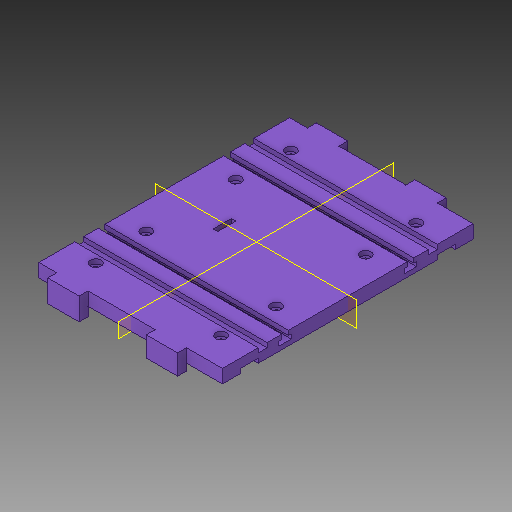
# Autodesk Inventor part: BandSawJigBottom
Saved by Autodesk Inventor 2019 (Build 230136000, 136)
## iProperties
Created: 2017-12-10
Part Number: BandSawJigBottom
Material: LCP Plastic
Document SubType Name: Modeling
Designer: steele
Density: 1.626 g/cm^3
Appearance: Violet
Author: steele
Autodesk Inventor part; units mm, degrees
ref_plane "YZ Plane" through (0, 0, 0) normal (1, 0, 0) x (0, 1, 0)
ref_plane "XZ Plane" through (0, 0, 0) normal (0, 1, 0) x (-1, 0, 0)
sketch "Sketch3" plane through (0, 0, 0) normal (0, 0, 1) x (1, 0, 0)
  line L0 (0, -9.525) -> (9.525, -9.525)
  line L1 (9.525, -9.525) -> (9.525, 0)
  line L2 (0, 0) -> (0, -9.525) construction
  line L3 (0, 0) -> (9.525, 0) construction
  line L4 (0, -9.525) -> (-9.525, -9.525)
  line L5 (-9.525, -9.525) -> (-9.525, 0)
  line L6 (9.525, 0) -> (73.025, 0)
  line L7 (-187.325, 0) -> (-187.325, 19.05)
  line L8 (-187.325, 0) -> (-9.525, 0)
  line L9 (73.025, 0) -> (73.025, 19.05)
  line L10 (73.025, 19.05) -> (-187.325, 19.05)
  dimension "d0" = 9.525
  dimension "d1" = 9.525
  dimension "d6" = 63.5
  dimension "d8" = 19.05
  dimension "d9" = 177.8
  constraints: 22 end point, 4 horizontal, 3 perpendicular, 2 symmetric about line, 1 vertical
  measures "d0" distance of L0.end L1.end
  measures "d1" distance of L0.start L0.end
  measures "d6" distance of L1.end L6.end
  measures "d8" distance of L6.end L9.end
  measures "d9" distance of L7.start L5.end
extrude "Extrusion1" add sketch "Sketch3" along normal mid plane 355.6
sketch "Sketch4" plane through (0, 0, 177.8) normal (0, 0, 1) x (1, 0, 0)
  line L0 (-187.325, 19.05) -> (73.025, 19.05) construction
  line L1 (0, 19.05) -> (0, -9.525) construction
  line L2 (9.525, -9.525) -> (-9.525, -9.525) construction
  line L3 (0, -9.525) -> (-22.225, -9.525)
  line L4 (-22.225, -9.525) -> (-22.225, 19.05)
  line L5 (-22.225, 19.05) -> (0, 19.05)
  line L6 (187.325, 19.05) -> (-73.025, 19.05) construction
  line L7 (0, -9.525) -> (22.225, -9.525)
  line L8 (22.225, -9.525) -> (22.225, 19.05)
  line L9 (0, 19.05) -> (22.225, 19.05)
  point P0 (0, 0)
  dimension "d12" = 22.225
  constraints: 16 end point, 4 point on line, 4 symmetric about line, 2 collinear, 1 midpoint, 1 perpendicular
  measures "d12" distance of L1.end L3.end
extrude "Extrusion2" add sketch "Sketch4" along normal blind 12.7
mirror "Mirror1" about plane through (0, 0, 0) normal (0, 0, 1) of "Extrusion2"
sketch "Sketch6" plane through (-187.325, 0, -177.8) normal (0, -1, 0) x (1, 0, 0)
  line L0 (82.55, 165.1) -> (88.9, 165.1)
  line L1 (88.9, 165.1) -> (88.9, 190.5)
  line L2 (88.9, 190.5) -> (82.55, 190.5)
  line L3 (82.55, 190.5) -> (82.55, 165.1)
  line L4 (82.55, 165.1) -> (88.9, 190.5) construction
  line L5 (88.9, 165.1) -> (82.55, 190.5) construction
  line L6 (177.8, 0) -> (177.8, 355.6) projected
  point P0 (187.325, 177.8)
  point P1 (85.725, 177.8)
  dimension "d16" = 12.7
  dimension "d18" = 6.35
  dimension "d19" = 88.9
  constraints: 12 end point, 2 midpoint, 2 parallel, 1 horizontal, 1 perpendicular
  measures "d16" distance from line of L2 point (85.725, 177.8)
  measures "d18" distance of L1.end L2.end
  measures "d19" distance between parallel lines of L1 L6
extrude "Extrusion3" cut sketch "Sketch6" against normal through all
sketch "Sketch7" plane through (0, 0, 177.8) normal (0, 0, 1) x (1, 0, 0)
  line L0 (-187.325, 19.05) -> (-22.225, 19.05) projected
  line L1 (-161.925, 19.05) -> (-117.475, 19.05)
  line L2 (-117.475, 19.05) -> (-117.475, -12.7)
  line L3 (-117.475, -12.7) -> (-161.925, -12.7)
  line L4 (-161.925, -12.7) -> (-161.925, 19.05)
  line L5 (-187.325, 19.05) -> (-187.325, 0) projected
  point P0 (0, 0)
  dimension "d22" = 44.45
  dimension "d23" = 31.75
  dimension "d24" = 25.4
  constraints: 8 end point, 2 parallel, 1 horizontal, 1 perpendicular, 1 point on line
  measures "d22" distance of L2.end L3.end
  measures "d23" distance of L1.end L2.end
  measures "d24" distance between parallel lines of L4 L5
extrude "Extrusion4" add sketch "Sketch7" along normal blind 12.7
mirror "Mirror2" about plane through (0, 0, 0) normal (0, 0, 1) of "Extrusion4"
sketch "Sketch9" plane through (73.025, 0, 177.8) normal (1, 0, 0) x (0, 0, -1)
  line L0 (355.6, 19.05) -> (0, 19.05) projected
  line L1 (50.8, 19.05) -> (63.5, 19.05)
  line L2 (63.5, 19.05) -> (63.5, 12.7)
  line L3 (63.5, 12.7) -> (50.8, 12.7)
  line L4 (50.8, 12.7) -> (50.8, 19.05)
  line L5 (0, 0) -> (0, 19.05) projected
  point P0 (177.8, 0)
  dimension "d28" = 12.7
  dimension "d29" = 6.35
  dimension "d30" = 50.8
  constraints: 8 end point, 2 parallel, 1 horizontal, 1 perpendicular, 1 point on line
  measures "d28" distance of L2.end L3.end
  measures "d29" distance of L1.end L2.end
  measures "d30" distance between parallel lines of L4 L5
extrude "Extrusion5" cut sketch "Sketch9" against normal through all
mirror "Mirror3" about plane through (0, 0, 0) normal (0, 0, 1) of "Extrusion5"
sketch "Sketch12" plane through (73.025, 0, 177.8) normal (1, 0, 0) x (0, 0, -1)
  line L0 (355.6, 0) -> (0, 0) construction
  line L1 (88.9, 0) -> (88.9, 16.5009) construction
  line L2 (0, 0) -> (0, 19.05) projected
  line L3 (50.8, 19.05) -> (0, 19.05) projected
  line L4 (84.1375, 19.05) -> (84.1375, 12.7)
  line L5 (84.1375, 12.7) -> (80.1624, 12.7)
  line L6 (80.1624, 12.7) -> (80.1624, 6.35)
  line L7 (80.1624, 6.35) -> (88.9, 6.35)
  line L8 (93.6625, 19.05) -> (93.6625, 12.7)
  line L9 (93.6625, 12.7) -> (97.6376, 12.7)
  line L10 (97.6376, 12.7) -> (97.6376, 6.35)
  line L11 (97.6376, 6.35) -> (88.9, 6.35)
  line L12 (84.1375, 19.05) -> (93.6625, 19.05)
  point P0 (177.8, 0)
  dimension "d46" = 88.9
  dimension "d47" = 4.7625
  dimension "d48" = 6.35
  dimension "d49" = 6.35
  dimension "d50" = 8.7376
  constraints: 20 end point, 4 symmetric about line, 3 point on line, 3 vertical, 1 collinear, 1 horizontal, 1 perpendicular
  measures "d46" distance between parallel lines of L1 L2
  measures "d47" distance between parallel lines of L4 L1
  measures "d48" distance of L4.start L4.end
  measures "d49" distance of L5.end L6.end
  measures "d50" distance of L6.end L7.end
extrude "Extrusion8" cut sketch "Sketch12" against normal through all
mirror "Mirror4" about plane through (0, 0, 0) normal (0, 0, 1) of "Extrusion8"
ref_plane "Work Plane1" through (-57.15, 0, 177.8) normal (1, 0, 0) x (0, 0, -1)
sketch "Sketch13" plane through (-57.15, 0, 177.8) normal (1, 0, 0) x (0, 0, -1)
  line L0 (25.4, 0) -> (50.8, 0)
  line L1 (50.8, 0) -> (50.8, 6.35)
  line L2 (50.8, 6.35) -> (25.4, 6.35)
  line L3 (25.4, 6.35) -> (25.4, 0)
  line L4 (0, 0) -> (0, 19.05) projected
  point P0 (177.8, 0)
  dimension "d54" = 25.4
  dimension "d55" = 6.35
  dimension "d56" = 25.4
  constraints: 8 end point, 2 parallel, 1 horizontal, 1 perpendicular
  measures "d54" distance of L0.start L0.end
  measures "d55" distance of L2.end L0.start
  measures "d56" distance between parallel lines of L4 L3
extrude "Extrusion9" cut sketch "Sketch13" along normal mid plane 260.35
mirror "Mirror5" about plane through (0, 0, 0) normal (0, 0, 1) of "Extrusion9"
sketch "Sketch14" plane through (0, 0, 0) normal (0, 0, 1) x (1, 0, 0)
  line L0 (-187.325, 0) -> (-161.925, 0) projected
  line L1 (-161.925, 0) -> (-136.525, 0)
  line L2 (-136.525, 0) -> (-136.525, 6.35)
  line L3 (-136.525, 6.35) -> (-161.925, 6.35)
  line L4 (-161.925, 6.35) -> (-161.925, 0)
  line L5 (-187.325, 19.05) -> (-187.325, 0) projected
  point P0 (0, 0)
  dimension "d59" = 25.4
  dimension "d60" = 6.35
  dimension "d61" = 25.4
  constraints: 8 end point, 2 parallel, 1 horizontal, 1 perpendicular, 1 point on line
  measures "d59" distance of L3.end L2.end
  measures "d60" distance of L2.end L1.end
  measures "d61" distance between parallel lines of L5 L4
extrude "Extrusion10" cut sketch "Sketch14" along normal mid plane 228.6
mirror "Mirror6" about plane through (-57.15, 0, 177.8) normal (1, 0, 0) of "Extrusion10"
sketch "Sketch16" plane through (-161.925, 6.35, -80.1624) normal (0, -1, 0) x (1, 0, 0)
  circle A0 centre (12.7, 143.6624) radius 3.3782
  line L0 (0, 194.4624) -> (25.4, 194.4624) projected
  line L1 (0, -34.1376) -> (0, 194.4624) projected
  point P0 (161.925, 80.1624)
  dimension "d71" = 6.7564
  dimension "d72" = 50.8
  dimension "d73" = 12.7
  constraints: 1 centre point
  measures "d71" diameter of A0
  measures "d72" distance from line of L0 A0.centre
  measures "d73" distance from line of A0.centre L1
extrude "Extrusion11" cut sketch "Sketch16" against normal through all
sketch "Sketch17" plane through (-187.325, 19.05, 84.1375) normal (0, 1, 0) x (1, 0, 0)
  circle A0 centre (38.1, 20.6375) radius 3.3782 projected
  circle A1 centre (38.1, 20.6375) radius 7.62
  point P0 (187.325, 84.1375)
  dimension "d76" = 15.24
  constraints: 1 centre point, 1 coincident
  measures "d76" diameter of A1
extrude "Extrusion12" cut sketch "Sketch17" against normal blind 6.35
mirror "Mirror7" about plane through (0, 0, 0) normal (0, 0, 1) of "Extrusion12", "Extrusion11"
mirror "Mirror8" about plane through (-57.15, 0, 177.8) normal (1, 0, 0) of "Extrusion12", "Extrusion11", "Mirror7"
sketch "Sketch18" plane through (-171.45, 6.35, 152.4) normal (0, -1, 0) x (1, 0, 0)
  circle A0 centre (203.2, -14.094) radius 3.3782
  line L0 (228.6, 0) -> (228.6, -25.4) projected
  point P0 (171.45, -152.4)
  dimension "d79" = 6.7564
  dimension "d80" = 25.4
  constraints: 1 centre point
  measures "d79" diameter of A0
  measures "d80" distance from line of L0 A0.centre
extrude "Extrusion13" cut sketch "Sketch18" against normal through all
sketch "Sketch19" plane through (22.225, 19.05, 177.8) normal (0, 1, 0) x (1, 0, 0)
  circle A0 centre (9.525, 39.494) radius 3.3782 projected
  circle A1 centre (9.525, 39.494) radius 7.62
  point P0 (-22.225, 177.8)
  dimension "d83" = 15.24
  constraints: 1 centre point, 1 coincident
  measures "d83" diameter of A1
extrude "Extrusion14" cut sketch "Sketch19" against normal blind 6.35
mirror "Mirror9" about plane through (-57.15, 0, 177.8) normal (1, 0, 0) of "Extrusion13", "Extrusion14"
mirror "Mirror10" about plane through (0, 0, 0) normal (0, 0, 1) of "Extrusion14", "Extrusion13", "Mirror9"
equation "\"d10\" = length"
equation "\"width\" = 260.35"
equation "\"length\" = 355.6"
equation "\"d53\" = -0.5 * width"
body "Solid1"
